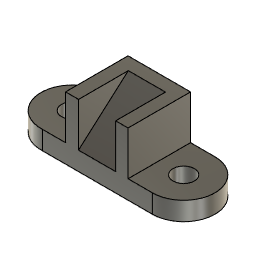
A3 v1 (Autodesk Fusion 360 design; units mm, degrees)
Autodesk Fusion 360 part; units mm, degrees
sketch "Base Sketch" plane through (0, 0, 0) normal (0, 0, 1) x (1, 0, 0)
  line L0 (57, 32) -> (-57, 32)
  line L1 (-57, -32) -> (57, -32)
  circle A0 centre (57, 0) radius 11
  circle A1 centre (-57, 0) radius 11.0308
  arc A2 (-55.5967, 32) -> (-55.5967, -32) centre (-57, 0) ccw
  arc A3 (57, -32) -> (57, 32) centre (57, 0) ccw
  dimension "d1" = 114
  dimension "d2" = 64
  dimension "d3" = 64.0615
  constraint horizontal L0
  constraint parallel L0 L1
  constraint coincident L1 A2.end
  constraint coincident L0 A2.start
  measures "d1" distance of L1.start L1.end
  measures "d2" distance of L0.end L1.start
  measures "d3" diameter of A2
extrude "Extrude1" add sketch "Base Sketch" along normal blind 19
sketch "Cube Sketch" plane through (0, 0, 19) normal (0, 0, 1) x (-1, 0, 0)
  circle A0 centre (57, 0) radius 11.0308
  circle A1 centre (-57, 0) radius 11
  arc A2 (-57, 32) -> (-57, -32) centre (-57, 0) ccw
  line L0 (-57, -32) -> (55.5967, -32)
  arc A3 (55.5967, -32) -> (55.5967, 32) centre (57, 0) ccw
  line L1 (55.5967, 32) -> (-57, 32)
  line L2 (32, 32) -> (-32, 32)
  line L3 (-32, 32) -> (-32, -32)
  line L4 (-32, -32) -> (32, -32)
  line L5 (32, -32) -> (32, 32)
  line L6 (32, 32) -> (-32, -32) construction
  line L7 (-32, 32) -> (32, -32) construction
  line L8 (18.7079, 32) -> (-19.2921, 32)
  line L9 (-19.2921, 32) -> (-19.2921, -19)
  line L10 (-19.2921, -19) -> (18.7079, -19)
  line L11 (18.7079, -19) -> (18.7079, 32)
  dimension "d8" = 64
  dimension "d9" = 64
  dimension "d10" = 38
  dimension "d11" = 51
  constraint horizontal L2
  constraint perpendicular L2 L3
  constraint parallel L2 L4
  constraint parallel L3 L5
  constraint coincident L6 origin
  constraint coincident L7 origin
  constraint horizontal L8
  constraint vertical L9
  constraint horizontal L10
  constraint vertical L11
  constraint coincident L2 L8.start
  measures "d8" distance of L3.end L4.end
  measures "d9" distance of L2.end L3.end
  measures "d10" distance of L8.start L8.end
  measures "d11" distance of L8.start L10.end
sketch "Triangle Sketch" plane through (0, 0, 0) normal (1, 0, 0) x (0, 1, 0)
  line L0 (-32, 19) -> (19, 19)
  line L1 (19, 19) -> (19, 64)
  line L2 (19, 64) -> (-32, 19)
  dimension "d12" = 51
  dimension "d13" = 45
  constraint horizontal L0
  constraint perpendicular L0 L1
  measures "d12" distance of L0.start L0.end
  measures "d13" distance of L0.end L1.end
extrude "Extrude2" add sketch "Triangle Sketch" along normal mid plane 38
extrude "Extrude3" add sketch "Cube Sketch" along normal blind 45 contours L0 L1 L2 L3 L4 L5 L9 L10 L11
equation "d2 = ( 32 * 2 ) * 1 mm"
equation "d13 = 64 mm - 19 mm"
